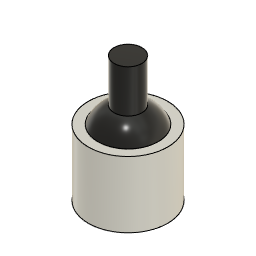
Ball Socket (Autodesk Fusion 360 design; units mm, degrees)
Autodesk Fusion 360 part; units mm, degrees
sphere "SpherePrimitive1" add diameter 50 placed x (1, 0, 0) y (0, 1, 0) z (0, 0, 1) at (0, 0, 0) makes body 1
move_body "MoveFace1" bodies 1 to x (1, 0, 0) y (0, 1, 0) z (0, 0, 1) at (0, 0, 25) on bodies 1
cylinder "CylinderPrimitive1" add diameter 21 height 80 placed x (1, 0, 0) y (0, 1, 0) z (0, 0, 1) at (0, 0, 0) bodies 1
delete_face "DeleteFace1" 1 faces at (10.4869, -0.5234, 1.5413) on bodies 1
cylinder "CylinderPrimitive2" add diameter 60 height 50 placed x (1, 0, 0) y (0, 1, 0) z (0, 0, 1) at (-0.9391, -55.4875, 0) separate body makes body 2
sphere "SpherePrimitive2" add diameter 50 placed x (1, 0, 0) y (0, 1, 0) z (0, 0, 1) at (-64.612, -128.6098, 0) separate body makes body 3
move_body "Move1" bodies 3 to x (1, 0, 0) y (0, 1, 0) z (0, 0, 1) at (63.6729, 73.1223, 50)
move_body "MoveFace2" bodies 3 to x (1, 0, 0) y (0, 1, 0) z (0, 0, 1) at (0, 0, -10) on bodies 3
combine "Combine1" operation cut target body 2 tool bodies 3
move_face "MoveFace3" to x (1, 0, 0) y (0, 1, 0) z (0, 0, 1) at (0, -10, 0) 2 faces at (20.6834, -67.9712, 38.725) (28.9118, -52.5004, 16.6667) on bodies 2
copy_body "Body->Comp1" bodies 1 removing the originals makes body 4 in component "Component"
copy_body "Body->Comp2" bodies 2 removing the originals makes body 5 in component "Component'"
move_body "Move1'" bodies 4 to x (1, 0, 0) y (0, 1, 0) z (0, 0, 1) at (0, 66, 0) in component "Component"
move_body "Move1''" bodies 5 to x (1, 0, 0) y (0, 1, 0) z (0, 0, 1) at (0, 66, 0) in component "Component'"
component "Component" placed x (1, 0, 0) y (0, 1, 0) z (0, 0, 1) at (-0.9391, -65.4875, 15)
component "Component'" placed x (1, 0, 0) y (0, 1, 0) z (0, 0, 1) at (0, 0, 0)
